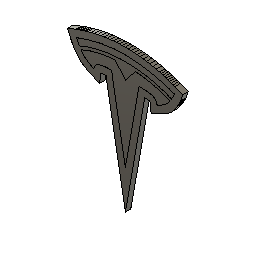
Tesla Logo (Autodesk Fusion 360 design; units mm, degrees)
Autodesk Fusion 360 part; units mm, degrees
note: some values were not read from the file. Chosen so that the rebuilt part matches the saved one: that a step has no effect; which pieces of a blend or face edit are solid. Set by a fixed rule: which sketch regions a step uses.
sketch "teslat" plane through (0, 0, 0) normal (0, 0, 1) x (1, 0, 0)
  line L0 (58.2836, 86.3887) -> (58.7276, 86.2696)
  line L1 (62.3187, 83.1899) -> (62.4168, 82.8531)
  line L2 (61.0882, 85.0852) -> (61.3274, 84.8611)
  line L3 (59.1435, 86.1387) -> (59.5319, 85.9957)
  line L4 (62.2027, 83.5093) -> (62.3187, 83.1899)
  line L5 (63.258, 82.0141) -> (63.7016, 82.2142)
  line L6 (63.7016, 82.2142) -> (64.2362, 82.4686)
  line L7 (59.5319, 85.9957) -> (59.8936, 85.8402)
  line L8 (65.5245, 83.1419) -> (66.2509, 83.5616)
  line L9 (57.3084, 86.5934) -> (57.8108, 86.4965)
  line L10 (62.5618, 82.126) -> (62.6102, 81.735)
  line L11 (62.9192, 81.8678) -> (63.258, 82.0141)
  line L12 (66.6287, 83.7925) -> (67.014, 84.0373)
  line L13 (69.3876, 85.8045) -> (69.7776, 86.1492)
  line L14 (66.2509, 83.5616) -> (66.6287, 83.7925)
  line L15 (69.7776, 86.1492) -> (70.1615, 86.5083)
  line L16 (53.6321, 86.9679) -> (54.3272, 86.9282)
  line L17 (61.9138, 84.098) -> (62.068, 83.8119)
  line L18 (70.1615, 86.5083) -> (70.5376, 86.882)
  line L19 (62.6102, 81.735) -> (62.9192, 81.8678)
  line L20 (58.7276, 86.2696) -> (59.1435, 86.1387)
  line L21 (68.5959, 85.1583) -> (68.9931, 85.4742)
  line L22 (68.1977, 84.8567) -> (68.5959, 85.1583)
  line L23 (67.4051, 84.2963) -> (67.8002, 84.5694)
  line L24 (62.4975, 82.4986) -> (62.5618, 82.126)
  line L25 (60.5399, 85.4901) -> (60.826, 85.2947)
  line L26 (70.5376, 86.882) -> (70.9041, 87.2702)
  line L27 (49.622, 87.0529) -> (51.3358, 87.0401)
  line L28 (67.014, 84.0373) -> (67.4051, 84.2963)
  line L29 (68.9931, 85.4742) -> (69.3876, 85.8045)
  line L30 (70.9041, 87.2702) -> (71.2594, 87.6731)
  line L31 (71.2594, 87.6731) -> (71.6018, 88.0906)
  line L32 (60.826, 85.2947) -> (61.0882, 85.0852)
  line L33 (9.8158, 85.8056) -> (10.2102, 85.4753)
  line L34 (53.2901, 94.4506) -> (52.5047, 94.5592)
  line L35 (22.3876, 93.8581) -> (21.4213, 93.6649)
  line L36 (58.778, 93.4504) -> (57.782, 93.6636)
  line L37 (56.2119, 86.7561) -> (56.7757, 86.6798)
  line L38 (9.3206, 90.0012) -> (8.1437, 89.5022)
  line L39 (51.7619, 94.6539) -> (50.4135, 94.8057)
  line L40 (29.9408, 94.9152) -> (28.7897, 94.807)
  line L41 (51.3358, 87.0401) -> (52.1371, 87.0235)
  line L42 (61.5442, 84.6222) -> (61.7395, 84.3679)
  line L43 (62.068, 83.8119) -> (62.2027, 83.5093)
  line L44 (71.9296, 88.5229) -> (72.241, 88.97)
  line L45 (61.7395, 84.3679) -> (61.9138, 84.098)
  line L46 (27.4412, 94.6553) -> (26.6985, 94.5605)
  line L47 (61.9215, 92.6811) -> (60.8499, 92.9602)
  line L48 (32.2225, 95.0734) -> (31.5813, 95.0331)
  line L49 (47.6218, 95.0317) -> (47.1676, 95.0575)
  line L50 (52.9023, 86.9996) -> (53.6321, 86.9679)
  line L51 (10.492, 90.4692) -> (9.3206, 90.0012)
  line L52 (28.7897, 94.807) -> (27.4412, 94.6553)
  line L53 (6.9636, 88.9712) -> (7.2747, 88.5241)
  line L54 (16.1897, 92.3792) -> (15.0787, 92.0512)
  line L55 (12.8095, 91.3162) -> (11.6557, 90.9072)
  line L56 (24.2227, 94.1889) -> (23.3222, 94.0325)
  line L57 (71.0607, 89.5011) -> (69.8837, 90.0001)
  line L58 (59.8936, 85.8402) -> (60.2294, 85.6718)
  line L59 (50.4135, 94.8057) -> (49.2623, 94.9139)
  line L60 (67.5484, 90.906) -> (66.3945, 91.315)
  line L61 (68.7122, 90.4681) -> (67.5484, 90.906)
  line L62 (56.7757, 86.6798) -> (57.3084, 86.5934)
  line L63 (9.042, 86.5094) -> (9.4258, 86.1503)
  line L64 (54.9884, 86.8799) -> (55.6164, 86.8226)
  line L65 (63.014, 92.378) -> (61.9215, 92.6811)
  line L66 (64.8484, 82.7777) -> (65.5245, 83.1419)
  line L67 (54.3272, 86.9282) -> (54.9884, 86.8799)
  line L68 (56.8157, 93.8569) -> (55.8811, 94.0312)
  line L69 (64.2362, 82.4686) -> (64.8484, 82.7777)
  line L70 (54.1162, 94.3271) -> (53.2901, 94.4506)
  line L71 (15.0787, 92.0512) -> (13.9512, 91.6972)
  line L72 (61.3274, 84.8611) -> (61.5442, 84.6222)
  line L73 (10.2102, 85.4753) -> (10.6073, 85.1595)
  line L74 (67.8002, 84.5694) -> (68.1977, 84.8567)
  line L75 (60.2294, 85.6718) -> (60.5399, 85.4901)
  line L76 (55.6164, 86.8226) -> (56.2119, 86.7561)
  line L77 (62.4168, 82.8531) -> (62.4975, 82.4986)
  line L78 (57.8108, 86.4965) -> (58.2836, 86.3887)
  line L79 (64.1251, 92.05) -> (63.014, 92.378)
  line L80 (49.2623, 94.9139) -> (48.3259, 94.9865)
  line L81 (47.1676, 95.0575) -> (46.9807, 95.072)
  line L82 (71.6018, 88.0906) -> (71.9296, 88.5229)
  line L83 (52.1371, 87.0235) -> (52.9023, 86.9996)
  line L84 (39.6099, 30.7442) -> (49.622, 87.0529)
  line L85 (66.3945, 91.315) -> (65.2526, 91.696)
  line L86 (20.4254, 93.4517) -> (19.4021, 93.2175)
  line L87 (14.9676, 82.4698) -> (15.5024, 82.2154)
  line L88 (19.4021, 93.2175) -> (18.3536, 92.9614)
  line L89 (55.8811, 94.0312) -> (54.9806, 94.1876)
  line L90 (47.5025, 97.3763) -> (48.5228, 97.2854)
  line L91 (20.9073, 86.3915) -> (21.3777, 86.4996)
  line L92 (44.4837, 97.5737) -> (45.4827, 97.5202)
  line L93 (18.1143, 85.0868) -> (18.3757, 85.2964)
  line L94 (21.8776, 86.5968) -> (22.4074, 86.6834)
  line L95 (9.4258, 86.1503) -> (9.8158, 85.8056)
  line L96 (15.5024, 82.2154) -> (16.285, 81.8689)
  line L97 (24.8419, 86.9332) -> (25.5328, 86.9734)
  line L98 (18.3757, 85.2964) -> (18.6607, 85.4919)
  line L99 (7.9445, 87.6742) -> (8.2997, 87.2713)
  line L100 (25.5328, 86.9734) -> (26.2581, 87.0055)
  line L101 (17.6595, 84.6236) -> (17.8758, 84.8627)
  line L102 (40.5651, 97.6731) -> (41.5327, 97.6648)
  line L103 (39.606, 97.671) -> (40.5651, 97.6731)
  line L104 (19.3046, 85.8423) -> (19.6648, 85.998)
  line L105 (8.6661, 86.8831) -> (9.042, 86.5094)
  line L106 (30.8772, 94.9879) -> (29.9408, 94.9152)
  line L107 (39.6099, 86.0753) -> (32.2225, 95.0734)
  line L108 (7.6023, 88.0918) -> (7.9445, 87.6742)
  line L109 (17.1367, 83.8132) -> (17.2907, 84.0993)
  line L110 (51.6228, 96.9323) -> (52.6685, 96.7868)
  line L111 (69.8837, 90.0001) -> (68.7122, 90.4681)
  line L112 (54.9806, 94.1876) -> (54.1162, 94.3271)
  line L113 (8.1437, 89.5022) -> (6.9636, 88.9712)
  line L114 (20.0515, 86.1411) -> (20.4654, 86.2722)
  line L115 (25.0871, 94.3283) -> (24.2227, 94.1889)
  line L116 (11.403, 84.5706) -> (11.7982, 84.2974)
  line L117 (10.6073, 85.1595) -> (11.0055, 84.8579)
  line L118 (57.782, 93.6636) -> (56.8157, 93.8569)
  line L119 (23.3222, 94.0325) -> (22.3876, 93.8581)
  line L120 (48.3259, 94.9865) -> (47.6218, 95.0317)
  line L121 (46.9807, 95.072) -> (39.5933, 86.0742)
  line L122 (59.8013, 93.2163) -> (58.778, 93.4504)
  line L123 (31.5813, 95.0331) -> (30.8772, 94.9879)
  line L124 (8.2997, 87.2713) -> (8.6661, 86.8831)
  line L125 (60.8499, 92.9602) -> (59.8013, 93.2163)
  line L126 (41.5327, 97.6648) -> (42.5085, 97.6457)
  line L127 (21.4213, 93.6649) -> (20.4254, 93.4517)
  line L128 (25.9131, 94.4519) -> (25.0871, 94.3283)
  line L129 (18.3536, 92.9614) -> (17.2821, 92.6823)
  line L130 (48.5228, 97.2854) -> (49.5498, 97.1813)
  line L131 (26.6985, 94.5605) -> (25.9131, 94.4519)
  line L132 (22.9681, 86.76) -> (23.5603, 86.8269)
  line L133 (65.2526, 91.696) -> (64.1251, 92.05)
  line L134 (17.4647, 84.3693) -> (17.6595, 84.6236)
  line L135 (11.6557, 90.9072) -> (10.492, 90.4692)
  line L136 (16.5941, 81.7361) -> (16.6427, 82.1272)
  line L137 (52.5047, 94.5592) -> (51.7619, 94.6539)
  line L138 (13.9512, 91.6972) -> (12.8095, 91.3162)
  line L139 (52.6685, 96.7868) -> (53.7199, 96.6268)
  line L140 (46.489, 97.4545) -> (47.5025, 97.3763)
  line L141 (24.1846, 86.8845) -> (24.8419, 86.9332)
  line L142 (17.2821, 92.6823) -> (16.1897, 92.3792)
  line L143 (72.241, 88.97) -> (71.0607, 89.5011)
  line L144 (39.5933, 86.0742) -> (39.6099, 86.0753)
  line L145 (26.2581, 87.0055) -> (27.0185, 87.03)
  line L146 (49.5498, 97.1813) -> (50.5832, 97.0637)
  line L147 (53.7199, 96.6268) -> (54.7769, 96.4521)
  line L148 (7.2747, 88.5241) -> (7.6023, 88.0918)
  line L149 (17.8758, 84.8627) -> (18.1143, 85.0868)
  line L150 (66.9559, 97.951) -> (65.7737, 98.2943)
  line L151 (18.9701, 85.6738) -> (19.3046, 85.8423)
  line L152 (17.2907, 84.0993) -> (17.4647, 84.3693)
  line L153 (57.6788, 100.2263) -> (56.55, 100.4387)
  line L154 (60.1375, 95.3445) -> (61.2233, 95.0739)
  line L155 (70.036, 92.2646) -> (71.1501, 91.8278)
  line L156 (52.1107, 101.1413) -> (51.0205, 101.2818)
  line L157 (62.2645, 99.2209) -> (61.1078, 99.4962)
  line L158 (55.4287, 100.6361) -> (54.3149, 100.8188)
  line L159 (46.7434, 101.7121) -> (45.6958, 101.7883)
  line L160 (45.6958, 101.7883) -> (44.6572, 101.8526)
  line L161 (43.6277, 101.9053) -> (42.6076, 101.9466)
  line L162 (39.6045, 102.0059) -> (38.6133, 101.9966)
  line L163 (56.55, 100.4387) -> (55.4287, 100.6361)
  line L164 (65.7737, 98.2943) -> (64.5976, 98.6202)
  line L165 (38.6133, 101.9966) -> (37.6123, 101.977)
  line L166 (57.979, 95.8356) -> (59.056, 95.5982)
  line L167 (12.5746, 83.7936) -> (12.9525, 83.5628)
  line L168 (16.788, 82.8543) -> (16.8861, 83.1911)
  line L169 (58.8147, 99.9987) -> (57.6788, 100.2263)
  line L170 (59.056, 95.5982) -> (60.1375, 95.3445)
  line L171 (12.1893, 84.0385) -> (12.5746, 83.7936)
  line L172 (51.0205, 101.2818) -> (49.9385, 101.4088)
  line L173 (44.6572, 101.8526) -> (43.6277, 101.9053)
  line L174 (64.5038, 94.158) -> (65.6044, 93.8169)
  line L175 (37.6123, 101.977) -> (36.6017, 101.9466)
  line L176 (36.6017, 101.9466) -> (35.5816, 101.9053)
  line L177 (50.5832, 97.0637) -> (51.6228, 96.9323)
  line L178 (61.1078, 99.4962) -> (59.9578, 99.7554)
  line L179 (34.5522, 101.8526) -> (33.5136, 101.7883)
  line L180 (12.9525, 83.5628) -> (13.679, 83.143)
  line L181 (73.9276, 91.8942) -> (74.3677, 92.7459)
  line L182 (14.3552, 82.7788) -> (14.9676, 82.4698)
  line L183 (22.4074, 86.6834) -> (22.9681, 86.76)
  line L184 (41.5969, 101.977) -> (40.5958, 101.9966)
  line L185 (53.2088, 100.9871) -> (52.1107, 101.1413)
  line L186 (47.7998, 101.6236) -> (46.7434, 101.7121)
  line L187 (64.5976, 98.6202) -> (63.4278, 98.9289)
  line L188 (59.9578, 99.7554) -> (58.8147, 99.9987)
  line L189 (54.7769, 96.4521) -> (55.8392, 96.2621)
  line L190 (17.0021, 83.5106) -> (17.1367, 83.8132)
  line L191 (16.285, 81.8689) -> (16.5941, 81.7361)
  line L192 (11.0055, 84.8579) -> (11.403, 84.5706)
  line L193 (74.1689, 95.5076) -> (72.9532, 95.962)
  line L194 (16.8861, 83.1911) -> (17.0021, 83.5106)
  line L195 (13.679, 83.143) -> (14.3552, 82.7788)
  line L196 (21.3777, 86.4996) -> (21.8776, 86.5968)
  line L197 (18.6607, 85.4919) -> (18.9701, 85.6738)
  line L198 (23.5603, 86.8269) -> (24.1846, 86.8845)
  line L199 (43.4922, 97.6155) -> (44.4837, 97.5737)
  line L200 (45.4827, 97.5202) -> (46.489, 97.4545)
  line L201 (55.8392, 96.2621) -> (56.9066, 96.0567)
  line L202 (11.7982, 84.2974) -> (12.1893, 84.0385)
  line L203 (29.5171, 87.0611) -> (39.6099, 30.7442)
  line L204 (27.8146, 87.0471) -> (29.5171, 87.0611)
  line L205 (27.0185, 87.03) -> (27.8146, 87.0471)
  line L206 (19.6648, 85.998) -> (20.0515, 86.1411)
  line L207 (42.5085, 97.6457) -> (43.4922, 97.6155)
  line L208 (16.7071, 82.4998) -> (16.788, 82.8543)
  line L209 (20.4654, 86.2722) -> (20.9073, 86.3915)
  line L210 (63.4067, 94.481) -> (64.5038, 94.158)
  line L211 (56.9066, 96.0567) -> (57.979, 95.8356)
  line L212 (16.6427, 82.1272) -> (16.7071, 82.4998)
  line L213 (30.3447, 101.5226) -> (29.2711, 101.4087)
  line L214 (4.9161, 92.6219) -> (5.3327, 91.8097)
  line L215 (67.8148, 93.079) -> (68.9241, 92.6815)
  line L216 (37.6777, 97.6648) -> (38.6454, 97.6731)
  line L217 (28.6267, 97.0637) -> (29.6601, 97.1813)
  line L218 (5.8262, 90.8937) -> (6.944, 91.371)
  line L219 (5.3327, 91.8097) -> (5.8262, 90.8937)
  line L220 (15.8028, 94.481) -> (16.8964, 94.7862)
  line L221 (19.0719, 95.3445) -> (20.1534, 95.5982)
  line L222 (16.946, 99.2207) -> (15.7828, 98.9288)
  line L223 (8.6737, 96.8132) -> (7.4687, 96.3971)
  line L224 (25.4898, 96.6268) -> (26.5413, 96.7868)
  line L225 (3.8224, 95.0336) -> (3.944, 94.7316)
  line L226 (48.8649, 101.5226) -> (47.7998, 101.6236)
  line L227 (74.3677, 92.7459) -> (74.7145, 93.4543)
  line L228 (9.174, 92.2646) -> (10.2857, 92.6815)
  line L229 (12.5015, 93.4573) -> (13.6052, 93.8169)
  line L230 (9.8732, 97.2107) -> (8.6737, 96.8132)
  line L231 (74.7145, 93.4543) -> (74.9776, 94.0247)
  line L232 (20.1534, 95.5982) -> (21.2305, 95.8356)
  line L233 (13.4371, 98.2942) -> (12.2551, 97.9509)
  line L234 (6.944, 91.371) -> (8.06, 91.8278)
  line L235 (14.6131, 98.6201) -> (13.4371, 98.2942)
  line L236 (61.2233, 95.0739) -> (62.3131, 94.7862)
  line L237 (75.292, 94.773) -> (75.3895, 95.0336)
  line L238 (42.6076, 101.9466) -> (41.5969, 101.977)
  line L239 (54.3149, 100.8188) -> (53.2088, 100.9871)
  line L240 (63.4278, 98.9289) -> (62.2645, 99.2209)
  line L241 (69.338, 97.2108) -> (68.1441, 97.5899)
  line L242 (65.6044, 93.8169) -> (66.7081, 93.4573)
  line L243 (74.9776, 94.0247) -> (75.292, 94.773)
  line L244 (70.5377, 96.8133) -> (69.338, 97.2108)
  line L245 (71.1501, 91.8278) -> (72.2663, 91.371)
  line L246 (73.3843, 90.8937) -> (73.9276, 91.8942)
  line L247 (26.001, 100.987) -> (24.895, 100.8187)
  line L248 (66.7081, 93.4573) -> (67.8148, 93.079)
  line L249 (68.9241, 92.6815) -> (70.036, 92.2646)
  line L250 (29.6601, 97.1813) -> (30.6872, 97.2854)
  line L251 (32.7211, 97.4545) -> (33.7275, 97.5202)
  line L252 (4.0903, 94.385) -> (4.2986, 93.9145)
  line L253 (14.7057, 94.158) -> (15.8028, 94.481)
  line L254 (71.7428, 96.3971) -> (70.5377, 96.8133)
  line L255 (31.4097, 101.6236) -> (30.3447, 101.5226)
  line L256 (68.1441, 97.5899) -> (66.9559, 97.951)
  line L257 (7.4687, 96.3971) -> (6.2584, 95.962)
  line L258 (72.2663, 91.371) -> (73.3843, 90.8937)
  line L259 (28.1892, 101.2817) -> (27.0991, 101.1412)
  line L260 (32.4661, 101.712) -> (31.4097, 101.6236)
  line L261 (75.3895, 95.0336) -> (74.1689, 95.5076)
  line L262 (35.7181, 97.6155) -> (36.7019, 97.6457)
  line L263 (38.6454, 97.6731) -> (39.6045, 97.671)
  line L264 (62.3131, 94.7862) -> (63.4067, 94.481)
  line L265 (29.2711, 101.4087) -> (28.1892, 101.2817)
  line L266 (72.9532, 95.962) -> (71.7428, 96.3971)
  line L267 (2.2003, 87.4509) -> (2.0096, 87.3128)
  line L268 (35.5816, 101.9053) -> (34.5522, 101.8526)
  line L269 (49.9385, 101.4088) -> (48.8649, 101.5226)
  line L270 (27.0991, 101.1412) -> (26.001, 100.987)
  line L271 (23.3704, 96.2621) -> (24.4327, 96.4521)
  line L272 (40.5958, 101.9966) -> (39.6045, 102.0059)
  line L273 (10.2857, 92.6815) -> (11.395, 93.079)
  line L274 (33.5136, 101.7883) -> (32.4661, 101.712)
  line L275 (17.9862, 95.0739) -> (19.0719, 95.3445)
  line L276 (16.8964, 94.7862) -> (17.9862, 95.0739)
  line L277 (4.1343, 84.4353) -> (4.6051, 83.9013)
  line L278 (75.9747, 85.5824) -> (76.3437, 86.1121)
  line L279 (74.598, 83.8994) -> (75.0688, 84.4332)
  line L280 (75.5286, 84.9939) -> (75.9747, 85.5824)
  line L281 (11.395, 93.079) -> (12.5015, 93.4573)
  line L282 (34.7266, 97.5737) -> (35.7181, 97.6155)
  line L283 (77.0018, 87.4421) -> (77.7782, 88.5076)
  line L284 (77.7782, 88.5076) -> (78.3461, 89.5532)
  line L285 (6.0614, 82.4509) -> (6.578, 81.9943)
  line L286 (30.6872, 97.2854) -> (31.7076, 97.3763)
  line L287 (78.3461, 89.5532) -> (78.8348, 90.499)
  line L288 (72.6527, 82.0155) -> (73.6073, 82.8835)
  line L289 (57.5285, 81.4052) -> (57.6169, 81.3727)
  line L290 (22.3029, 96.0567) -> (23.3704, 96.2621)
  line L291 (3.6746, 84.9962) -> (4.1343, 84.4353)
  line L292 (23.7813, 100.636) -> (22.6601, 100.4386)
  line L293 (13.6052, 93.8169) -> (14.7057, 94.158)
  line L294 (39.6293, 2.292) -> (53.7929, 81.9487)
  line L295 (57.0794, 81.535) -> (57.3286, 81.4681)
  line L296 (15.7828, 98.9288) -> (14.6131, 98.6201)
  line L297 (36.7019, 97.6457) -> (37.6777, 97.6648)
  line L298 (21.2305, 95.8356) -> (22.3029, 96.0567)
  line L299 (56.4345, 81.6698) -> (56.7812, 81.603)
  line L300 (11.067, 97.5898) -> (9.8732, 97.2107)
  line L301 (19.2525, 99.7553) -> (18.1027, 99.4961)
  line L302 (3.2286, 85.5849) -> (3.6746, 84.9962)
  line L303 (12.2551, 97.9509) -> (11.067, 97.5898)
  line L304 (39.6045, 97.671) -> (39.606, 97.671)
  line L305 (74.1184, 83.3914) -> (74.598, 83.8994)
  line L306 (9.4648, 79.8449) -> (10.3788, 79.2752)
  line L307 (18.1027, 99.4961) -> (16.946, 99.2207)
  line L308 (73.6073, 82.8835) -> (74.1184, 83.3914)
  line L309 (8.06, 91.8278) -> (9.174, 92.2646)
  line L310 (26.5413, 96.7868) -> (27.587, 96.9323)
  line L311 (21.5314, 100.2262) -> (20.3955, 99.9986)
  line L312 (20.3955, 99.9986) -> (19.2525, 99.7553)
  line L313 (14.2861, 77.2858) -> (20.7348, 74.5154)
  line L314 (69.7387, 79.8439) -> (70.6899, 80.4877)
  line L315 (68.8249, 79.2743) -> (69.7387, 79.8439)
  line L316 (25.3529, 81.9528) -> (39.6293, 2.292)
  line L317 (4.6051, 83.9013) -> (5.0846, 83.3931)
  line L318 (21.5881, 81.3783) -> (21.675, 81.4105)
  line L319 (4.5726, 93.3251) -> (4.9161, 92.6219)
  line L320 (27.587, 96.9323) -> (28.6267, 97.0637)
  line L321 (11.2424, 78.7763) -> (12.0429, 78.3452)
  line L322 (5.0429, 95.5076) -> (3.8224, 95.0336)
  line L323 (6.2584, 95.962) -> (5.0429, 95.5076)
  line L324 (22.6601, 100.4386) -> (21.5314, 100.2262)
  line L325 (77.1921, 87.3034) -> (77.0018, 87.4421)
  line L326 (12.7668, 77.9797) -> (13.4161, 77.6709)
  line L327 (22.4148, 81.6076) -> (22.7584, 81.6744)
  line L328 (3.944, 94.7316) -> (4.0903, 94.385)
  line L329 (4.2986, 93.9145) -> (4.5726, 93.3251)
  line L330 (22.1194, 81.5397) -> (22.4148, 81.6076)
  line L331 (12.0429, 78.3452) -> (12.7668, 77.9797)
  line L332 (24.895, 100.8187) -> (23.7813, 100.636)
  line L333 (33.7275, 97.5202) -> (34.7266, 97.5737)
  line L334 (24.4327, 96.4521) -> (25.4898, 96.6268)
  line L335 (5.5707, 82.91) -> (6.0614, 82.4509)
  line L336 (2.0096, 87.3128) -> (2.8598, 86.1148)
  line L337 (56.0696, 81.729) -> (56.4345, 81.6698)
  line L338 (2.8598, 86.1148) -> (3.2286, 85.5849)
  line L339 (64.9186, 77.2849) -> (65.8171, 77.6827)
  line L340 (31.7076, 97.3763) -> (32.7211, 97.4545)
  line L341 (72.1401, 101.5497) -> (70.881, 101.9668)
  line L342 (5.8068, 101.1129) -> (4.5371, 100.6564)
  line L343 (10.3788, 79.2752) -> (11.2424, 78.7763)
  line L344 (65.8171, 77.6827) -> (67.1373, 78.3314)
  line L345 (-0.6692, 92.8022) -> (-0.2521, 91.841)
  line L346 (57.6169, 81.3727) -> (58.4662, 74.512)
  line L347 (71.6657, 81.2098) -> (72.6527, 82.0155)
  line L348 (26.4315, 106.0968) -> (24.1138, 105.7576)
  line L349 (5.0846, 83.3931) -> (5.5707, 82.91)
  line L350 (79.9402, 92.9279) -> (81.8024, 97.9071)
  line L351 (74.6744, 100.6565) -> (73.4046, 101.113)
  line L352 (23.12, 81.7335) -> (24.0759, 81.8525)
  line L353 (22.7584, 81.6744) -> (23.12, 81.7335)
  line L354 (70.6899, 80.4877) -> (71.6657, 81.2098)
  line L355 (6.578, 81.9943) -> (7.5374, 81.2111)
  line L356 (58.4662, 74.512) -> (64.9186, 77.2849)
  line L357 (52.7782, 106.0969) -> (50.494, 106.3781)
  line L358 (33.1772, 106.7772) -> (30.9646, 106.604)
  line L359 (7.0711, 101.5495) -> (5.8068, 101.1129)
  line L360 (16.9735, 104.3673) -> (14.5358, 103.7712)
  line L361 (59.8268, 104.8956) -> (57.446, 105.3581)
  line L362 (81.8024, 97.9071) -> (75.9493, 100.18)
  line L363 (25.1762, 81.9438) -> (25.3529, 81.9528)
  line L364 (76.3437, 86.1121) -> (77.1921, 87.3034)
  line L365 (79.2307, 91.308) -> (79.5538, 92.0084)
  line L366 (78.8348, 90.499) -> (79.2307, 91.308)
  line L367 (13.4161, 77.6709) -> (14.2861, 77.2858)
  line L368 (8.5134, 80.4888) -> (9.4648, 79.8449)
  line L369 (41.7214, 106.9757) -> (39.6045, 107.0064)
  line L370 (21.675, 81.4105) -> (21.8727, 81.4731)
  line L371 (39.6045, 107.0064) -> (37.4878, 106.9757)
  line L372 (79.5538, 92.0084) -> (79.9402, 92.9279)
  line L373 (21.7639, 105.358) -> (19.3834, 104.8954)
  line L374 (73.4046, 101.113) -> (72.1401, 101.5497)
  line L375 (30.9646, 106.604) -> (28.7155, 106.3781)
  line L376 (19.3834, 104.8954) -> (16.9735, 104.3673)
  line L377 (55.096, 105.7577) -> (52.7782, 106.0969)
  line L378 (24.0759, 81.8525) -> (25.1762, 81.9438)
  line L379 (50.494, 106.3781) -> (48.2449, 106.6041)
  line L380 (0.9069, 89.4827) -> (1.4243, 88.5223)
  line L381 (21.8727, 81.4731) -> (22.1194, 81.5397)
  line L382 (7.5374, 81.2111) -> (8.5134, 80.4888)
  line L383 (57.3286, 81.4681) -> (57.5285, 81.4052)
  line L384 (1.4243, 88.5223) -> (2.2003, 87.4509)
  line L385 (28.7155, 106.3781) -> (26.4315, 106.0968)
  line L386 (0.4349, 90.4028) -> (0.9069, 89.4827)
  line L387 (53.998, 81.9384) -> (55.1066, 81.8477)
  line L388 (14.5358, 103.7712) -> (12.0868, 103.1086)
  line L389 (12.0868, 103.1086) -> (10.8308, 102.7438)
  line L390 (43.8572, 106.9003) -> (41.7214, 106.9757)
  line L391 (56.7812, 81.603) -> (57.0794, 81.535)
  line L392 (67.9614, 78.7753) -> (68.8249, 79.2743)
  line L393 (67.1373, 78.3314) -> (67.9614, 78.7753)
  line L394 (3.2624, 100.1799) -> (-2.7068, 97.8618)
  line L395 (70.881, 101.9668) -> (69.6276, 102.3648)
  line L396 (-0.2521, 91.841) -> (0.4349, 90.4028)
  line L397 (55.1066, 81.8477) -> (56.0696, 81.729)
  line L398 (57.446, 105.3581) -> (55.096, 105.7577)
  line L399 (75.0688, 84.4332) -> (75.5286, 84.9939)
  line L400 (67.1386, 103.1045) -> (65.9032, 103.4468)
  line L401 (4.5371, 100.6564) -> (3.2624, 100.1799)
  line L402 (20.7348, 74.5154) -> (21.5881, 81.3783)
  line L403 (75.9493, 100.18) -> (74.6744, 100.6565)
  line L404 (53.7929, 81.9487) -> (53.998, 81.9384)
  line L405 (68.3801, 102.744) -> (67.1386, 103.1045)
  line L406 (8.3301, 101.9667) -> (7.0711, 101.5495)
  line L407 (35.3521, 106.9003) -> (33.1772, 106.7772)
  line L408 (69.6276, 102.3648) -> (68.3801, 102.744)
  line L409 (48.2449, 106.6041) -> (46.0321, 106.7773)
  line L410 (9.5833, 102.3647) -> (8.3301, 101.9667)
  line L411 (64.6597, 103.775) -> (62.2368, 104.3675)
  line L412 (24.1138, 105.7576) -> (21.7639, 105.358)
  line L413 (62.2368, 104.3675) -> (59.8268, 104.8956)
  line L414 (-2.7068, 97.8618) -> (-0.6692, 92.8022)
  line L415 (46.0321, 106.7773) -> (43.8572, 106.9003)
  line L416 (37.4878, 106.9757) -> (35.3521, 106.9003)
  line L417 (10.8308, 102.7438) -> (9.5833, 102.3647)
  line L418 (65.9032, 103.4468) -> (64.6597, 103.775)
extrude "Extrude1" add sketch "teslat" against normal blind 1 contours L0 L1 L2 L3 L4 L5 L6 L7 L8 L9 L10 L11 L12 L13 L14 L15 L16 L17 L18 L19 L20 L21 L22 L23 L24 L25 L26 L27 L28 L29 L30 L31 L32 L33 L34 L35 L36 L37 L38 L39 L40 L41 L42 L43 L44 L45 L46 L47 L48 L49 L50 L51 L52 L53 L54 L55 L56 L57 L58 L59 L60 L61 L62 L63 L64 L65 L66 L67 L68 L69 L70 L71 L72 L73 L74 L75 L76 L77 L78 L79 L80 L81 L82 L83 L84 L85 L86 L87 L88 L89 L91 L93 L94 L95 L96 L97 L98 L99 L100 L101 L104 L105 L106 L107 L108 L109 L111 L112 L113 L114 L115 L116 L117 L118 L119 L120 L121 L122 L123 L124 L125 L127 L128 L129 L131 L132 L133 L134 L135 L136 L137 L138 L141 L142 L143 L145 L148 L149 L151 L152 L167 L168 L171 L180 L182 L183 L190 L191 L192 L194 L195 L196 L197 L198 L202 L203 L204 L205 L206 L208 L209 L212 | L90 L92 L102 L103 L110 L126 L130 L139 L140 L146 L147 L150 L153 L154 L155 L156 L157 L158 L159 L160 L161 L162 L163 L164 L165 L166 L169 L170 L172 L173 L174 L175 L176 L177 L178 L179 L181 L184 L185 L186 L187 L188 L189 L193 L199 L200 L201 L207 L210 L211 L213 L214 L215 L216 L217 L218 L219 L220 L221 L222 L223 L224 L225 L226 L227 L228 L229 L230 L231 L232 L233 L234 L235 L236 L237 L238 L239 L240 L241 L242 L243 L244 L245 L246 L247 L248 L249 L250 L251 L252 L253 L254 L255 L256 L257 L258 L259 L260 L261 L262 L263 L264 L265 L266 L268 L269 L270 L271 L272 L273 L274 L275 L276 L281 L282 L286 L290 L292 L293 L296 L297 L298 L300 L301 L303 L307 L309 L310 L311 L312 L319 L320 L322 L323 L324 L328 L329 L332 L333 L334 L340 | L267 L277 L278 L279 L280 L283 L284 L285 L287 L288 L289 L291 L294 L295 L299 L302 L305 L306 L308 L313 L314 L315 L316 L317 L318 L321 L325 L326 L327 L330 L331 L335 L336 L337 L338 L339 L341 L342 L343 L344 L345 L346 L347 L348 L349 L350 L351 L352 L353 L354 L355 L356 L357 L358 L359 L360 L361 L362 L363 L364 L365 L366 L367 L368 L369 L370 L371 L372 L373 L374 L375 L376 L377 L378 L379 L380 L381 L382 L383 L384 L385 L386 L387 L388 L389 L390 L391 L392 L393 L394 L395 L396 L397 L398 L399 L400 L401 L402 L403 L404 L405 L406 L407 L408 L409 L410 L411 L412 L413 L414 L415 L416 L417 L418 makes body 1
extrude "Extrude2" add sketch "teslat" along normal blind 3 separate body contours L0 L1 L2 L3 L4 L5 L6 L7 L8 L9 L10 L11 L12 L13 L14 L15 L16 L17 L18 L19 L20 L21 L22 L23 L24 L25 L26 L27 L28 L29 L30 L31 L32 L33 L34 L35 L36 L37 L38 L39 L40 L41 L42 L43 L44 L45 L46 L47 L48 L49 L50 L51 L52 L53 L54 L55 L56 L57 L58 L59 L60 L61 L62 L63 L64 L65 L66 L67 L68 L69 L70 L71 L72 L73 L74 L75 L76 L77 L78 L79 L80 L81 L82 L83 L84 L85 L86 L87 L88 L89 L91 L93 L94 L95 L96 L97 L98 L99 L100 L101 L104 L105 L106 L107 L108 L109 L111 L112 L113 L114 L115 L116 L117 L118 L119 L120 L121 L122 L123 L124 L125 L127 L128 L129 L131 L132 L133 L134 L135 L136 L137 L138 L141 L142 L143 L145 L148 L149 L151 L152 L167 L168 L171 L180 L182 L183 L190 L191 L192 L194 L195 L196 L197 L198 L202 L203 L204 L205 L206 L208 L209 L212 | L90 L92 L102 L103 L110 L126 L130 L139 L140 L146 L147 L150 L153 L154 L155 L156 L157 L158 L159 L160 L161 L162 L163 L164 L165 L166 L169 L170 L172 L173 L174 L175 L176 L177 L178 L179 L181 L184 L185 L186 L187 L188 L189 L193 L199 L200 L201 L207 L210 L211 L213 L214 L215 L216 L217 L218 L219 L220 L221 L222 L223 L224 L225 L226 L227 L228 L229 L230 L231 L232 L233 L234 L235 L236 L237 L238 L239 L240 L241 L242 L243 L244 L245 L246 L247 L248 L249 L250 L251 L252 L253 L254 L255 L256 L257 L258 L259 L260 L261 L262 L263 L264 L265 L266 L268 L269 L270 L271 L272 L273 L274 L275 L276 L281 L282 L286 L290 L292 L293 L296 L297 L298 L300 L301 L303 L307 L309 L310 L311 L312 L319 L320 L322 L323 L324 L328 L329 L332 L333 L334 L340 makes body 2 at (36.2401, 67.9598, 0) makes body 3 at (72.8237, 93.5119, 0)
extrude "Extrude3" add sketch "teslat" along normal blind 3 separate body contours L267 L277 L278 L279 L280 L283 L284 L285 L287 L288 L289 L291 L294 L295 L299 L302 L305 L306 L308 L313 L314 L315 L316 L317 L318 L321 L325 L326 L327 L330 L331 L335 L336 L337 L338 L339 L341 L342 L343 L344 L345 L346 L347 L348 L349 L350 L351 L352 L353 L354 L355 L356 L357 L358 L359 L360 L361 L362 L363 L364 L365 L366 L367 L368 L369 L370 L371 L372 L373 L374 L375 L376 L377 L378 L379 L380 L381 L382 L383 L384 L385 L386 L387 L388 L389 L390 L391 L392 L393 L394 L395 L396 L397 L398 L399 L400 L401 L402 L403 L404 L405 L406 L407 L408 L409 L410 L411 L412 L413 L414 L415 L416 L417 L418 makes body 4
combine "Combine1" operation add target body 4 tool bodies 1
delete_face "DeleteFace1" 1 faces at (2.0731, 87.3588, 1.6667) on bodies 4
delete_face "DeleteFace2" 1 faces at (77.1287, 87.3497, 0.3333) on bodies 4
form "Form1" [no effect]
